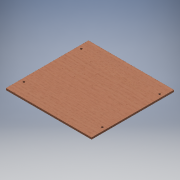
# Autodesk Inventor part: Wood Electronic  1
Saved by Autodesk Inventor 2019.4 (Build 234330000, 330)
## iProperties
Created: 2020-01-28
Part Number: Wood Electronic  1
Material: Wood (Oak)
Document SubType Name: Modeling
Designer: Mark
Mass: 226.67 g
Surface Area: 1241.86 cm^2
Volume: 298.25 cm^3
Density: 0.76 g/cm^3
Appearance: White Oak - Natural Medium Gloss
Author: Mark
Autodesk Inventor part; units mm, degrees
ref_plane "YZ Plane" through (0, 0, 0) normal (1, 0, 0) x (0, 1, 0)
ref_plane "XZ Plane" through (0, 0, 0) normal (0, 1, 0) x (-1, 0, 0)
ref_plane "XY Plane" through (0, 0, 0) normal (0, 0, 1) x (1, 0, 0)
sketch "Sketch1" plane through (0, 0, 0) normal (0, 1, 0) x (-1, 0, 0)
  line L0 (-119.3, 115) -> (119.3, 115)
  line L1 (119.3, 115) -> (119.3, -115)
  line L2 (119.3, -115) -> (-119.3, -115)
  line L3 (-119.3, -115) -> (-119.3, 115)
  line L4 (-119.3, 115) -> (119.3, -115) construction
  line L5 (119.3, 115) -> (-119.3, -115) construction
  point P0 (0, 0)
  dimension "d0" = 238.6
  dimension "d1" = 230
  constraints: 12 end point, 2 midpoint, 2 parallel, 1 horizontal, 1 perpendicular
  measures "d0" distance of L1.end L2.end
  measures "d1" distance of L0.end L1.end
extrude "Extrusion1" add sketch "Sketch1" along normal blind 5
sketch "Sketch3" plane through (0, 0, 0) normal (0, -1, 0) x (1, 0, 0)
  circle A0 centre (-109.3, 75) radius 2.75
  circle A1 centre (-109.3, -85) radius 2.75
  circle A2 centre (109.3, -85) radius 2.75
  circle A3 centre (109.3, 75) radius 2.75
  line L0 (119.3, -115) -> (119.3, 115) projected
  line L1 (-119.3, 115) -> (-119.3, -115) projected
  line L2 (119.3, 115) -> (-119.3, 115) projected
  line L3 (-119.3, -115) -> (119.3, -115) projected
  point P0 (0, 0)
  dimension "d11" = 5.5
  dimension "d12" = 5.5
  dimension "d13" = 5.5
  dimension "d14" = 5.5
  dimension "d15" = 10
  dimension "d16" = 10
  dimension "d17" = 10
  dimension "d18" = 10
  dimension "d19" = 40
  dimension "d20" = 40
  dimension "d21" = 30
  dimension "d22" = 30
  constraints: 4 centre point
  measures "d11" diameter of A0
  measures "d12" diameter of A1
  measures "d13" diameter of A2
  measures "d14" diameter of A3
  measures "d15" distance from line of L0 A3.centre
  measures "d16" distance from line of L0 A2.centre
  measures "d17" distance from line of L1 A1.centre
  measures "d18" distance from line of L1 A0.centre
  measures "d19" distance from line of L2 A0.centre
  measures "d20" distance from line of L2 A3.centre
  measures "d21" distance from line of L3 A2.centre
  measures "d22" distance from line of L3 A1.centre
extrude "Extrusion3" cut sketch "Sketch3" against normal blind 5 contours A0 | A1 | A2 | A3
body "Solid1"
